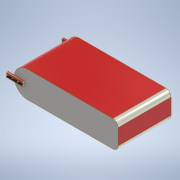
# Autodesk Inventor part: Battery_temp
Saved by Autodesk Inventor 2022 (Build 260153000, 153)
## iProperties
Created: 2023-01-30
Part Number: Battery_temp
Material: Generic
Document SubType Name: Modeling
Designer: scott
Density: 1 g/cm^3
Appearance: Titanium
Author: scott
Autodesk Inventor part; units mm, degrees
ref_plane "YZ Plane" through (0, 0, 0) normal (1, 0, 0) x (0, 1, 0)
ref_plane "XZ Plane" through (0, 0, 0) normal (0, 1, 0) x (-1, 0, 0)
ref_plane "XY Plane" through (0, 0, 0) normal (0, 0, 1) x (1, 0, 0)
sketch "Sketch2" plane through (0, 0, 0) normal (0, 0, 1) x (1, 0, 0)
  line L0 (-51.5, 15) -> (0, 15)
  line L1 (0, 15) -> (0, 0)
  line L2 (0, 0) -> (-51.5, 0)
  line L3 (-51.5, 0) -> (-51.5, 15)
  circle A0 centre (-51.5, 7.5) radius 7.5
  dimension "d0" = 15
  dimension "d1" = 0
  dimension "d2" = 51.5
  dimension "d3" = 0
  constraints: 8 end point, 2 parallel, 1 horizontal, 1 midpoint, 1 perpendicular, 3 other
  measures "d0" distance between parallel lines of L2 L0
  measures "d1" distance from line of point (0, 0) L2
  measures "d2" distance of L0.start L0.end
  measures "d3" distance from line of point (0, 0) L1
extrude "Extrusion1" add sketch "Sketch2" along normal blind 30
sketch "Sketch3" plane through (0, 0, 30) normal (0, 0, 1) x (1, 0, 0)
  line L0 (-53, 9) -> (-62, 9)
  line L1 (-62, 9) -> (-62, 6)
  line L2 (-62, 6) -> (-53, 6)
  line L3 (-53, 6) -> (-53, 9)
  line L4 (-51.5, 0) -> (0, 0) projected
  line L5 (0, 0) -> (0, 15) projected
  arc A0 (-51.5, 15) -> (-51.5, 0) centre (-51.5, 7.5) ccw projected
  dimension "d6" = 3
  dimension "d7" = 6
  dimension "d8" = 53
  dimension "d9" = 10.5
  constraints: 8 end point, 2 parallel, 1 horizontal, 1 perpendicular
  measures "d6" distance between parallel lines of L2 L0
  measures "d7" distance between parallel lines of L4 L2
  measures "d8" distance between parallel lines of L5 L3
  measures "d9" distance from line of A0.centre L1
extrude "Extrusion2" add sketch "Sketch3" along normal blind 1.5
sketch "Sketch4" plane through (-62, 6, 30) normal (-1, 0, 0) x (0, 0, 1)
  circle A0 centre (0.75, 2.25) radius 0.7503
  circle A1 centre (0.75, 0.75) radius 0.7524
  line L0 (0, 3) -> (1.5, 3) projected
  line L1 (0, 0) -> (1.5, 0) projected
  line L2 (0, 3) -> (0, 9) projected
  line L3 (1.5, 3) -> (1.5, 0) projected
  line L4 (0, 3) -> (1.5, 3)
  line L5 (1.5, 3) -> (1.5, 0)
  line L6 (1.5, 0) -> (0, 0)
  line L7 (0, 0) -> (0, 3)
  point P0 (-30, -6)
  point P1 (1.5, 2.2724)
  point P2 (0.7724, 3)
  point P3 (0, 2.2276)
  point P4 (0, 0.8104)
  point P5 (0.7045, 1.501)
  point P6 (0, 2.2724)
  point P7 (0.7276, 3)
  point P8 (1.5, 0.8104)
  point P9 (1.5, 2.2276)
  point P10 (0.7955, 1.501)
  point P11 (1.5, 0.6896)
  point P12 (0.8104, 0)
  point P13 (0, 0.6896)
  point P14 (0.6896, 0)
  dimension "d12" = 0.75
  dimension "d13" = 0.75
  constraints: 8 end point, 2 centre point, 2 parallel, 1 horizontal, 1 perpendicular
  measures "d12" distance from line of A0.centre L0
  measures "d13" distance from line of L1 A1.centre
extrude "Extrusion3" cut sketch "Sketch4" against normal through all contours L3 A1 A0 | A0 L0 L3 | A0 L7 L0 | A0 A1 L7 | L3 L1 A1 | A1 L1 L7 picked at (1.3379, 1.4108)
sketch "Sketch5" plane through (0, 0, 0) normal (0, 0, -1) x (-1, 0, 0)
  line L0 (53, 9.75) -> (62, 9.75)
  line L1 (62, 9.75) -> (62, 5.25)
  line L2 (62, 5.25) -> (53, 5.25)
  line L3 (53, 5.25) -> (53, 9.75)
  line L4 (0, 0) -> (0, 15) projected
  line L5 (51.5, 0) -> (0, 0) projected
  line L6 (62, 6.8104) -> (62, 7.501) projected
  dimension "d16" = 4.5
  dimension "d17" = 53
  dimension "d18" = 5.25
  dimension "d19" = 0
  constraints: 8 end point, 2 parallel, 1 horizontal, 1 perpendicular
  measures "d16" distance of L2.end L0.start
  measures "d17" distance between parallel lines of L3 L4
  measures "d18" distance between parallel lines of L5 L2
  measures "d19" distance between parallel lines of L6 L1
extrude "Extrusion4" add sketch "Sketch5" along normal blind 1.5
sketch "Sketch6" plane through (-62, 5.25, 0) normal (-1, 0, 0) x (0, 0, 1)
  circle A0 centre (-0.75, 3.75) radius 0.7504
  circle A1 centre (-0.75, 2.25) radius 0.7519
  circle A2 centre (-0.75, 0.75) radius 0.75
  line L0 (-1.5, 4.5) -> (-1.5, 0) projected
  line L1 (0, 4.5) -> (-1.5, 4.5) projected
  line L2 (-1.5, 4.5) -> (0, 4.5)
  line L3 (0, 4.5) -> (0, 0)
  line L4 (0, 0) -> (-1.5, 0)
  line L5 (-1.5, 0) -> (-1.5, 4.5)
  point P0 (0, -5.25)
  point P1 (-1.5, 3.7258)
  point P2 (-1.5, 2.304)
  point P3 (-0.7918, 3.0008)
  point P4 (-0.7742, 4.5)
  point P5 (-1.5, 3.7742)
  point P6 (0, 3.7742)
  point P7 (-0.7258, 4.5)
  point P8 (0, 2.304)
  point P9 (0, 3.7258)
  point P10 (-0.7082, 3.0008)
  point P11 (-0.75, 0)
  point P12 (0, 0.75)
  point P13 (-1.5, 0.75)
  point P14 (0, 2.196)
  point P15 (-0.7118, 1.499)
  point P16 (-1.5, 2.196)
  point P17 (-0.7882, 1.499)
  dimension "d22" = 1.5
  dimension "d23" = 0.75
  dimension "d24" = 0.75
  dimension "d25" = 1.5
  constraints: 8 end point, 3 centre point, 2 parallel, 1 horizontal, 1 perpendicular, 1 tangent
  measures "d22" distance of A1.centre A0.centre
  measures "d23" distance from line of L0 A0.centre
  measures "d24" distance from line of L1 A0.centre
  measures "d25" distance of A1.centre A2.centre
extrude "Extrusion5" cut sketch "Sketch6" against normal through all contours L3 A1 A0 | A0 L1 L3 | A0 L0 L1 | L3 A2 A1 | A0 A1 L0 | A2 L0 A1 | L3 L4 A2 | A2 L4 L0
fillet "Fillet1" radius 3 2 edges at (0, 15, 15) (0, 0, 15)
body "Solid1"
